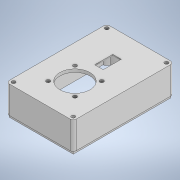
# Autodesk Inventor part: top
Saved by Autodesk Inventor 2020 (Build 240168000, 168)
## iProperties
Created: 2020-01-18
Part Number: top
Material: Generic
Document SubType Name: Modeling
Designer: chris
Density: 1 g/cm^3
Appearance: Default
Author: chris
Autodesk Inventor part; units mm, degrees
ref_plane "YZ Plane" through (0, 0, 0) normal (1, 0, 0) x (0, 1, 0)
ref_plane "XZ Plane" through (0, 0, 0) normal (0, 1, 0) x (-1, 0, 0)
ref_plane "XY Plane" through (0, 0, 0) normal (0, 0, 1) x (1, 0, 0)
sketch "Sketch2" plane through (35, 0, -52.5) normal (0, 1, 0) x (-1, 0, 0)
  line L0 (0, 0) -> (70, 0)
  line L1 (70, 0) -> (70, 105)
  line L2 (70, 105) -> (0, 105)
  line L3 (0, 105) -> (0, 0)
  dimension "d0" = 70
  dimension "d1" = 105
  constraints: 8 end point, 2 parallel, 1 horizontal, 1 perpendicular
  measures "d0" distance of L2.end L1.end
  measures "d1" distance of L1.end L0.end
extrude "Extrusion1" add sketch "Sketch2" along normal blind 3.175
sketch "Sketch3" plane through (35, 0, -52.5) normal (0, -1, 0) x (1, 0, 0)
  line L0 (-3.175, 101.825) -> (-66.825, 101.825)
  line L1 (-66.825, 101.825) -> (-66.825, 3.175)
  line L2 (-66.825, 3.175) -> (-3.175, 3.175)
  line L3 (-3.175, 3.175) -> (-3.175, 101.825)
  line L4 (0, 105) -> (0, 0) projected
  line L5 (-70, 0) -> (-70, 105) projected
  line L6 (0, 0) -> (-70, 0) projected
  line L7 (-70, 105) -> (0, 105) projected
  line L8 (-70, 105) -> (0, 105) projected
  line L9 (-70, 0) -> (-70, 105) projected
  line L10 (0, 105) -> (-70, 105)
  line L11 (-70, 105) -> (-70, 0)
  line L12 (-70, 0) -> (0, 0)
  line L13 (0, 0) -> (0, 105)
  point P0 (-35, 52.5)
  dimension "d5" = 3.175
  dimension "d6" = 3.175
  dimension "d7" = 3.175
  dimension "d8" = 3.175
  constraints: 16 end point, 4 parallel, 2 horizontal, 2 perpendicular
  measures "d5" distance between parallel lines of L3 L4
  measures "d6" distance between parallel lines of L5 L1
  measures "d7" distance between parallel lines of L6 L2
  measures "d8" distance between parallel lines of L0 L7
extrude "Extrusion2" add sketch "Sketch3" along normal blind 25.4
sketch "Sketch4" plane through (35, -25.4, -52.5) normal (0, -1, 0) x (1, 0, 0)
  line L0 (-1.5875, 103.4125) -> (-68.4125, 103.4125)
  line L1 (-68.4125, 103.4125) -> (-68.4125, 1.5875)
  line L2 (-68.4125, 1.5875) -> (-1.5875, 1.5875)
  line L3 (-1.5875, 1.5875) -> (-1.5875, 103.4125)
  line L4 (-3.175, 101.825) -> (-3.175, 3.175) projected
  line L5 (-3.175, 3.175) -> (-66.825, 3.175) projected
  line L6 (-3.175, 101.825) -> (-66.825, 101.825)
  line L7 (-66.825, 101.825) -> (-66.825, 3.175)
  line L8 (-66.825, 3.175) -> (-3.175, 3.175)
  line L9 (-3.175, 3.175) -> (-3.175, 101.825)
  line L10 (-3.175, 101.825) -> (-66.825, 101.825)
  line L11 (-66.825, 101.825) -> (-66.825, 3.175)
  line L12 (-66.825, 3.175) -> (-3.175, 3.175)
  line L13 (-3.175, 3.175) -> (-3.175, 101.825)
  point P0 (-35, 52.5)
  dimension "d11" = 1.5875
  dimension "d12" = 1.5875
  dimension "d13" = 1.5875
  dimension "d14" = 1.5875
  constraints: 24 end point, 6 parallel, 3 horizontal, 3 perpendicular
  measures "d11" distance between parallel lines of L4 L3
  measures "d12" distance between parallel lines of L2 L5
  measures "d13" distance between parallel lines of L1 L7
  measures "d14" distance between parallel lines of L0 L6
extrude "Extrusion3" add sketch "Sketch4" along normal blind 3.175
sketch "Sketch5" plane through (35, 0, -52.5) normal (0, -1, 0) x (1, 0, 0)
  line L0 (-3.175, 101.825) -> (-66.825, 101.825) projected
  line L1 (-3.175, 3.175) -> (-3.175, 101.825) projected
  arc A0 (-6.985, 101.825) -> (-3.175, 98.015) centre (-3.175, 101.825) ccw
  arc A1 (-3.175, 6.985) -> (-6.985, 3.175) centre (-3.175, 3.175) ccw
  line L2 (-66.825, 3.175) -> (-3.175, 3.175) projected
  arc A2 (-63.015, 3.175) -> (-66.825, 6.985) centre (-66.825, 3.175) ccw
  line L3 (-66.825, 101.825) -> (-66.825, 3.175) projected
  arc A3 (-66.825, 98.015) -> (-63.015, 101.825) centre (-66.825, 101.825) ccw
  line L4 (-3.175, 101.825) -> (-66.825, 101.825)
  line L5 (-66.825, 101.825) -> (-66.825, 3.175)
  line L6 (-66.825, 3.175) -> (-3.175, 3.175)
  line L7 (-3.175, 3.175) -> (-3.175, 101.825)
  point P0 (-35, 52.5)
  point P1 (-3.175, 6.985)
  dimension "d17" = 3.81
  constraints: 8 end point, 8 point on circle, 4 centre point, 3 equal radius, 2 coincident, 2 parallel, 2 point on line, 1 horizontal, 1 perpendicular
  measures "d17" radius of A0
extrude "Extrusion4" add sketch "Sketch5" along normal up to surface (28.575 mm away) contours L1 A0 L0 | A3 L3 L0 | L1 L2 A1 | A2 L2 L3
sketch "Sketch6" plane through (35, -28.575, -52.5) normal (0, -1, 0) x (1, 0, 0)
  circle A0 centre (-3.81, 101.19) radius 1.905
  line L0 (0, 0) -> (0, 105) projected
  line L1 (0, 105) -> (-70, 105) projected
  circle A1 centre (-3.81, 3.81) radius 1.905
  circle A2 centre (-66.19, 101.19) radius 1.905
  circle A3 centre (-66.19, 3.81) radius 1.905
  line L2 (-70, 0) -> (0, 0) projected
  line L3 (-70, 105) -> (-70, 0) projected
  point P0 (-35, 52.5)
  dimension "d20" = 3.81
  dimension "d21" = 3.81
  dimension "d22" = 3.81
  dimension "d23" = 3.81
  dimension "d24" = 3.81
  dimension "d25" = 3.81
  dimension "d26" = 3.81
  dimension "d27" = 3.81
  dimension "d28" = 3.81
  dimension "d29" = 3.81
  dimension "d30" = 3.81
  dimension "d31" = 3.81
  constraints: 4 centre point
  measures "d20" diameter of A0
  measures "d21" distance from line of L0 A0.centre
  measures "d22" distance from line of L1 A0.centre
  measures "d23" diameter of A1
  measures "d24" diameter of A2
  measures "d25" diameter of A3
  measures "d26" distance from line of L0 A1.centre
  measures "d27" distance from line of L2 A1.centre
  measures "d28" distance from line of L2 A3.centre
  measures "d29" distance from line of L3 A3.centre
  measures "d30" distance from line of L3 A2.centre
  measures "d31" distance from line of L1 A2.centre
extrude "Extrusion5" cut sketch "Sketch6" against normal through all contours A0 | A1 | A2 | A3
sketch "Sketch7" plane through (35, 0, -52.5) normal (0, -1, 0) x (1, 0, 0)
  circle A0 centre (-49, 54.2351) radius 2
  circle A1 centre (-49, 82.2351) radius 2
  circle A2 centre (-21, 54.2351) radius 2
  circle A3 centre (-21, 82.2351) radius 2
  line L0 (-49, 54.2351) -> (-21, 54.2351)
  line L1 (-21, 54.2351) -> (-21, 82.2351)
  line L2 (-21, 82.2351) -> (-49, 82.2351)
  line L3 (-49, 82.2351) -> (-49, 54.2351)
  line L4 (-49, 82.2351) -> (-70, 82.2351)
  line L5 (-70, 0) -> (-70, 105) projected
  line L6 (-21, 82.2351) -> (0, 82.2351)
  line L7 (0, 105) -> (0, 0) projected
  circle A4 centre (-35, 68.2351) radius 15.7055
  point P0 (-35, 52.5)
  dimension "d34" = 4
  dimension "d36" = 28
  dimension "d37" = 28
  constraints: 12 end point, 5 centre point, 4 coincident, 3 equal radius, 3 point on line, 2 horizontal, 2 parallel, 1 collinear, 1 perpendicular
  measures "d34" diameter of A0
  measures "d36" distance of L2.end L1.end
  measures "d37" distance of L1.end L0.end
extrude "Extrusion6" cut sketch "Sketch7" against normal through all contours L0 L3 A0 | A0 L3 L0 | A4 L3 L2 L1 L0 | L0 A4 | A4 L3 | L0 L1 A2 | A2 L1 L0 | L1 A4 | L3 L2 A1 | A1 L4 L3 | A4 L2 | A1 L2 L4 | L1 L6 A3 | A3 L2 L1 | A3 L6 L2
sketch "Sketch8" plane through (35, 3.175, -52.5) normal (0, 1, 0) x (1, 0, 0)
  circle A0 centre (-35, -68.0248) radius 40
  circle A1 centre (-35, -68.0248) radius 30
  line L0 (-39.445, -43.1383) -> (-30.555, -43.1383)
  line L1 (-30.555, -43.1383) -> (-30.555, -24.259)
  line L2 (-30.555, -24.259) -> (-39.445, -24.259)
  line L3 (-39.445, -24.259) -> (-39.445, -43.1383)
  line L4 (-39.445, -24.259) -> (-70, -24.259)
  line L5 (-70, 0) -> (-70, -105) projected
  line L6 (-30.555, -24.259) -> (0, -24.259)
  line L7 (0, 0) -> (0, -105) projected
  point P0 (-35, -52.5)
  dimension "d40" = 80
  dimension "d41" = 60
  dimension "d42" = 8.89
  constraints: 12 end point, 3 point on line, 2 centre point, 2 horizontal, 2 parallel, 1 coincident, 1 collinear, 1 perpendicular
  measures "d40" diameter of A0
  measures "d41" diameter of A1
  measures "d42" distance of L1.end L2.end
extrude "Extrusion7" cut sketch "Sketch8" against normal through all contours L1 A1 L3 A0 | A0 L3 L2 L1 | L1 L0 L3 A1 picked at (-35.4955, -41.4461)
fillet "Fillet2" radius 3.175 4 edges at (-35, -11.1125, -52.5) (-35, -11.1125, 52.5) (35, -11.1125, 52.5) (35, -11.1125, -52.5)
fillet "Fillet3" radius 3.175 8 edges at (0, 0, -49.325) (-31.825, 0, 0) (-29.1309, 0, -46.6309) (31.825, 0, 0) (0, 0, 49.325) (29.1309, 0, 46.6309) (-29.1309, 0, 46.6309) (29.1309, 0, -46.6309)
fillet "Fillet4" radius 3.175 4 edges at (0, 0, -28.241) (4.445, 0, -18.8013) (-4.445, 0, -18.8013) (0, 0, -9.3617)
body "Solid1"
